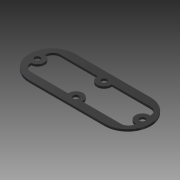
# Autodesk Inventor part: ConnectorSeal
Saved by Autodesk Inventor 2014 SP2 (Build 180246200, 246)
## iProperties
Created: 2015-09-19
Part Number: ConnectorSeal
Material: Rubber, Silicone
Document SubType Name: Modeling
Designer: Lukasz Szmit
Density: 1.25 g/cm^3
Appearance: Rubber - Black - Version 1.1
Author: Lukasz Szmit
Autodesk Inventor part; units mm, degrees
ref_plane "YZ Plane" through (0, 0, 0) normal (1, 0, 0) x (0, 1, 0)
ref_plane "XZ Plane" through (0, 0, 0) normal (0, 1, 0) x (-1, 0, 0)
ref_plane "XY Plane" through (0, 0, 0) normal (0, 0, 1) x (1, 0, 0)
sketch "Sketch1" plane through (0, 0, 0) normal (0, 0, 1) x (1, 0, 0)
  line L0 (-28, 17) -> (28, 17)
  line L1 (45, 0) -> (45, 0)
  line L2 (28, -17) -> (-28, -17)
  line L3 (-45, 0) -> (-45, 0)
  arc A0 (-28, 17) -> (-28, -17) centre (-28, 0) ccw
  arc A1 (28, -17) -> (28, 17) centre (28, 0) ccw
  point P0 (0, 0)
  point P1 (-45, 17)
  point P2 (45, 17)
  point P3 (-45, -17)
  dimension "d0" = 90
  dimension "d1" = 34
  dimension "d2" = 17
  dimension "d3" = 17
  dimension "d4" = 90
  dimension "d5" = 56
  dimension "d6" = 28
  constraints: 8 end point, 8 point on circle, 6 point on line, 4 tangent, 2 centre point, 2 perpendicular
  measures "d0" distance of point (-45, 17) point (45, 17)
  measures "d1" distance of point (-45, -17) point (-45, 17)
  measures "d2" distance from line of point (0, 0) L0
  measures "d3" radius of A0
  measures "d4" horizontal distance of point (45, 17) point (-45, -17)
  measures "d5" distance of A1.centre A0.centre
  measures "d6" distance of point (0, 0) A0.centre
sketch "Sketch2" plane through (0, 0, 0) normal (0, 0, 1) x (1, 0, 0)
  circle A0 centre (-39, 0) radius 2
  circle A1 centre (39, 0) radius 2
  circle A2 centre (0, -10.5) radius 2
  circle A3 centre (0, 10.5) radius 2
  point P0 (0, 0)
  point P1 (0, 0)
  point P2 (-3.3578, 23.5)
  dimension "d7" = 4
  dimension "d8" = 4
  dimension "d9" = 4
  dimension "d10" = 4
  dimension "d11" = 78
  dimension "d12" = 21
  dimension "d13" = 39
  constraints: 4 centre point
  measures "d7" diameter of A0
  measures "d8" diameter of A2
  measures "d9" diameter of A1
  measures "d10" diameter of A3
  measures "d11" distance of A1.centre A0.centre
  measures "d12" distance of A3.centre A2.centre
  measures "d13" horizontal distance of A1.centre A2.centre
sketch "Sketch3" plane through (0, 0, 0) normal (0, 0, 1) x (1, 0, 0)
  arc A0 (-5.2261, 11) -> (5.2261, 11) centre (0, 10.5) ccw
  arc A1 (-38.5, -5.2262) -> (-38.5, 5.2261) centre (-39, 0) ccw
  arc A2 (5.2261, -11) -> (-5.2261, -11) centre (0, -10.5) ccw
  arc A3 (39.5, 5.2261) -> (39.5, -5.2262) centre (39, 0) ccw
  line L0 (-38.5, -5.2262) -> (-38.5, -5.5)
  line L1 (-33, -11) -> (-5.2261, -11)
  line L2 (39.5, 5.2261) -> (39.5, 5.5)
  line L3 (34, 11) -> (5.2261, 11)
  line L4 (-5.2261, 11) -> (-33, 11)
  line L5 (-38.5, 5.5) -> (-38.5, 5.2261)
  line L6 (5.2261, -11) -> (34, -11)
  line L7 (39.5, -5.5) -> (39.5, -5.2262)
  arc A4 (-33, 11) -> (-38.5, 5.5) centre (-33, 5.5) ccw
  arc A5 (-38.5, -5.5) -> (-33, -11) centre (-33, -5.5) ccw
  arc A6 (39.5, 5.5) -> (34, 11) centre (34, 5.5) ccw
  arc A7 (34, -11) -> (39.5, -5.5) centre (34, -5.5) ccw
  point P0 (43.6422, -42)
  dimension "d14" = 5.5
  dimension "d15" = 5.25
  dimension "d16" = 5.25
  dimension "d17" = 5.25
  dimension "d18" = 5.25
  dimension "d19" = 22
  dimension "d20" = 78
  dimension "d23" = 5.5
  dimension "d24" = 5.5
  dimension "d25" = 5.5
  dimension "d26" = 78
  constraints: 16 end point, 16 point on circle, 8 centre point, 8 tangent, 3 equal radius, 1 coincident, 1 collinear
  measures "d14" radius of A4
  measures "d15" radius of A0
  measures "d16" radius of A1
  measures "d17" radius of A2
  measures "d18" radius of A3
  measures "d19" distance between parallel lines of L6 L3
  measures "d20" distance between parallel lines of L5 L2
  measures "d23" radius of A5
  measures "d24" radius of A7
  measures "d25" radius of A6
  measures "d26" distance of L7.end L0.start
extrude "Extrusion1" add sketch "Sketch1" along normal blind 1.5
extrude "Extrusion2" cut sketch "Sketch3" along normal blind 1.5
hole "Hole1" at (-39, 0, 0) at (0, 10.5, 0) at (0, -10.5, 0) at (39, 0, 0) direction (0, 0, 1) diameter 4 end through all
equation "\"d2\" = 0.5 * d1"
equation "\"d3\" = 0.5 * d1"
equation "\"d4\" = d0"
equation "\"d5\" = d0 - 2 * d3"
equation "\"d6\" = 0.5 * d5"
equation "\"d8\" = d7"
equation "\"d9\" = d7"
equation "\"d10\" = d7"
equation "\"d14\" = 0.5 * d21"
equation "\"d15\" = d16"
equation "\"d17\" = d16"
equation "\"d18\" = d16"
equation "\"d19\" = 2 * d21"
equation "\"d26\" = d20"
equation "\"d21\" = 11"
body "Solid1"
